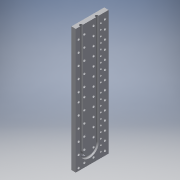
# Autodesk Inventor part: 17-0028-0016
Saved by Autodesk Inventor 2016 SP2 (Build 200236200, 236)
## iProperties
Category: IOP
Company: Universiteit van Amsterdam
RuleStatus: InUse
BeforeDocSave0: Open Form
Created: 2017-11-01
Part Number: 17-0028-0016
Material: Aluminum-6061
Document SubType Name: Modeling
Designer: Daan Giesen
Density: 2.71 g/cm^3
Appearance: Aluminum - Flat - Version 1.1
Mass: 501.104 g
Surface Area: 619.896 cm^2
Volume: 184.909 cm^3
Project: Digital PID Loop
Cost Center: 17-0028
User Status: CNC
Authority: Reichsöllner, Lukas
Description: Heat sink plate
Author: Daan Giesen
Title: Digital PID Loop
Revision Number: A.1
Autodesk Inventor part; units mm, degrees
ref_plane "YZ Plane" through (0, 0, 0) normal (1, 0, 0) x (0, 1, 0)
ref_plane "XZ Plane" through (0, 0, 0) normal (0, 1, 0) x (-1, 0, 0)
ref_plane "XY Plane" through (0, 0, 0) normal (0, 0, 1) x (1, 0, 0)
sketch "Sketch1" plane through (0, 0, 0) normal (0, 0, 1) x (1, 0, 0)
  line L0 (0, 52.5) -> (0, -52.5) construction
  line L1 (-7, 0) -> (7, 0) construction
  line L2 (-5, -37.5) -> (5, -37.5)
  line L3 (5, -37.5) -> (5, 37.5)
  line L4 (5, 37.5) -> (-5, 37.5)
  line L5 (-5, 37.5) -> (-5, -37.5)
  line L6 (-5, -37.5) -> (5, 37.5) construction
  line L7 (5, -37.5) -> (-5, 37.5) construction
  point P0 (0, 0)
  dimension "d0" = 75
  dimension "d1" = 10
  constraints: 12 end point, 2 midpoint, 2 parallel, 1 horizontal, 1 perpendicular
  measures "d0" distance of L2.end L3.end
  measures "d1" distance of L3.end L4.end
extrude "Extrusion1" add sketch "Sketch1" along normal mid plane 284
sketch "Sketch5" plane through (5, -37.5, 142) normal (1, 0, 0) x (0, 0, -1)
  circle A0 centre (154, 67) radius 1.621 projected
  circle A1 centre (154, 41) radius 1.621 projected
  circle A2 centre (174, 67) radius 1.621 projected
  circle A3 centre (174, 41) radius 1.621 projected
  circle A4 centre (194, 67) radius 1.621 projected
  circle A5 centre (194, 41) radius 1.621 projected
  circle A6 centre (214, 67) radius 1.621 projected
  circle A7 centre (214, 41) radius 1.621 projected
  circle A8 centre (234, 67) radius 1.621 projected
  circle A9 centre (234, 41) radius 1.621 projected
  circle A10 centre (254, 67) radius 1.621 projected
  circle A11 centre (254, 41) radius 1.621 projected
  circle A12 centre (274, 67) radius 1.621 projected
  circle A13 centre (274, 41) radius 1.621 projected
  line L0 (299.292, 35) -> (299.292, 75) projected
  line L1 (299.292, 75) -> (0, 75) projected
  line L2 (299.292, 35) -> (0, 35) projected
  circle A14 centre (148, 7) radius 1.621 projected
  circle A15 centre (174, 7) radius 1.621 projected
  circle A16 centre (196.3, 20) radius 1.621 projected
  circle A17 centre (200, 7) radius 1.621 projected
  circle A18 centre (222.3, 20) radius 1.621 projected
  circle A19 centre (226, 7) radius 1.621 projected
  circle A20 centre (248.3, 20) radius 1.621 projected
  circle A21 centre (252, 7) radius 1.621 projected
  circle A22 centre (274.3, 20) radius 1.621 projected
  circle A23 centre (278, 7) radius 1.621 projected
  circle A24 centre (20.3, 13.85) radius 0.7835 projected
  circle A25 centre (33.3, 13.85) radius 0.7835 projected
  circle A26 centre (46.3, 13.85) radius 0.7835 projected
  circle A27 centre (59.3, 13.85) radius 0.7835 projected
  circle A28 centre (72.3, 13.85) radius 0.7835 projected
  circle A29 centre (85.3, 13.85) radius 0.7835 projected
  circle A30 centre (98.3, 13.85) radius 0.7835 projected
  circle A31 centre (111.3, 13.85) radius 0.7835 projected
  circle A32 centre (124.3, 13.85) radius 0.7835 projected
  circle A33 centre (136.7, 25.15) radius 0.7835 projected
  circle A34 centre (157.6, 13.85) radius 0.7835 projected
  circle A35 centre (170.6, 13.85) radius 0.7835 projected
  circle A36 centre (183.6, 13.85) radius 0.7835 projected
  circle A37 centre (196.6, 13.85) radius 0.7835 projected
  circle A38 centre (209, 25.15) radius 0.7835 projected
  circle A39 centre (222.6, 13.85) radius 0.7835 projected
  circle A40 centre (235, 25.15) radius 0.7835 projected
  circle A41 centre (248.6, 13.85) radius 0.7835 projected
  circle A42 centre (261, 25.15) radius 0.7835 projected
  circle A43 centre (274, 25.15) radius 0.7835 projected
  circle A44 centre (261.6, 13.85) radius 0.7835 projected
  circle A45 centre (248, 25.15) radius 0.7835 projected
  circle A46 centre (235.6, 13.85) radius 0.7835 projected
  circle A47 centre (222, 25.15) radius 0.7835 projected
  circle A48 centre (209.6, 13.85) radius 0.7835 projected
  circle A49 centre (196, 25.15) radius 0.7835 projected
  circle A50 centre (170, 25.15) radius 0.7835 projected
  circle A51 centre (144.6, 13.85) radius 0.7835 projected
  circle A52 centre (123.7, 25.15) radius 0.7835 projected
  circle A53 centre (97.7, 25.15) radius 0.7835 projected
  circle A54 centre (71.7, 25.15) radius 0.7835 projected
  circle A55 centre (58.7, 25.15) radius 0.7835 projected
  circle A56 centre (45.7, 25.15) radius 0.7835 projected
  circle A57 centre (32.7, 25.15) radius 0.7835 projected
  circle A58 centre (19.7, 25.15) radius 0.7835 projected
  circle A59 centre (7.3, 13.85) radius 0.7835 projected
  line L3 (289.292, 0) -> (289.292, 30) projected
  line L4 (289.292, 30) -> (0, 30) projected
  line L5 (0, 0) -> (0, 30) projected
  line L6 (289.292, 0) -> (0, 0) projected
  circle A60 centre (84.7, 25.15) radius 0.7835 projected
  circle A61 centre (84.7, 25.15) radius 0.7835 projected
  circle A62 centre (20.3, 20) radius 1.621 projected
  circle A63 centre (24, 7) radius 1.621 projected
  circle A64 centre (46.3, 20) radius 1.621 projected
  circle A65 centre (50, 7) radius 1.621 projected
  circle A66 centre (72.3, 20) radius 1.621 projected
  circle A67 centre (76, 7) radius 1.621 projected
  circle A68 centre (98.3, 20) radius 1.621 projected
  circle A69 centre (102, 7) radius 1.621 projected
  circle A70 centre (124.3, 20) radius 1.621 projected
  circle A71 centre (128, 7) radius 1.621 projected
  circle A72 centre (110.7, 25.15) radius 0.7835 projected
  circle A73 centre (110.7, 25.15) radius 0.7835 projected
  circle A74 centre (144, 20) radius 1.621 projected
  circle A75 centre (144.3, 20) radius 1.621 projected
  circle A76 centre (157, 25.15) radius 0.7835 projected
  circle A77 centre (157, 25.15) radius 0.7835 projected
  circle A78 centre (170, 20) radius 1.621 projected
  circle A79 centre (170.3, 20) radius 1.621 projected
  circle A80 centre (183, 25.15) radius 0.7835 projected
  circle A81 centre (183, 25.15) radius 0.7835 projected
  circle A82 centre (258.35, 57.639) radius 1.6 projected
  circle A83 centre (232.35, 57.639) radius 1.6 projected
  circle A84 centre (206.35, 57.639) radius 1.6 projected
  circle A85 centre (180.35, 57.639) radius 1.6 projected
  circle A86 centre (154.35, 57.639) radius 1.6 projected
  circle A87 centre (167.35, 57.639) radius 1.6 projected
  circle A88 centre (193.35, 57.639) radius 1.6 projected
  circle A89 centre (219.35, 57.639) radius 1.6 projected
  circle A90 centre (245.35, 57.639) radius 1.6 projected
  circle A91 centre (271.35, 57.639) radius 1.6 projected
  circle A92 centre (14, 67) radius 1.621 projected
  circle A93 centre (14, 41) radius 1.621 projected
  circle A94 centre (34, 67) radius 1.621 projected
  circle A95 centre (34, 41) radius 1.621 projected
  circle A96 centre (54, 67) radius 1.621 projected
  circle A97 centre (54, 41) radius 1.621 projected
  circle A98 centre (74, 67) radius 1.621 projected
  circle A99 centre (74, 41) radius 1.621 projected
  circle A100 centre (94, 67) radius 1.621 projected
  circle A101 centre (94, 41) radius 1.621 projected
  circle A102 centre (114, 67) radius 1.621 projected
  circle A103 centre (114, 41) radius 1.621 projected
  circle A104 centre (134, 67) radius 1.621 projected
  circle A105 centre (134, 41) radius 1.621 projected
  circle A106 centre (121.05, 57.639) radius 1.6 projected
  circle A107 centre (95.05, 57.639) radius 1.6 projected
  circle A108 centre (69.05, 57.639) radius 1.6 projected
  circle A109 centre (43.05, 57.639) radius 1.6 projected
  circle A110 centre (17.05, 57.639) radius 1.6 projected
  circle A111 centre (30.05, 57.639) radius 1.6 projected
  circle A112 centre (56.05, 57.639) radius 1.6 projected
  circle A113 centre (82.05, 57.639) radius 1.6 projected
  circle A114 centre (108.05, 57.639) radius 1.6 projected
  circle A115 centre (134.05, 57.639) radius 1.6 projected
  line L7 (0, 35) -> (0, 75) projected
  point P0 (142, 37.5)
  point P1 (274, 67)
  point P2 (254, 67)
  point P3 (274, 41)
  point P4 (194, 67)
  point P5 (174, 67)
  point P6 (174, 41)
  point P7 (154, 41)
  point P8 (134, 67)
  point P9 (134, 41)
  point P10 (114, 41)
  point P11 (94, 41)
  point P12 (94, 67)
  point P13 (54, 67)
  point P14 (34, 41)
  point P15 (34, 67)
  point P16 (14, 67)
  point P17 (274.3, 20)
  point P18 (252, 7)
  point P19 (222.3, 20)
  point P20 (226, 7)
  point P21 (196.3, 20)
  point P22 (200, 7)
  point P23 (144.3, 20)
  point P24 (148, 7)
  point P25 (124.3, 20)
  point P26 (128, 7)
  point P27 (72.3, 20)
  point P28 (76, 7)
  point P29 (24, 7)
  point P30 (20.3, 20)
  constraints: 36 coincident
hole "Hole1" at (5, -17.5, -132.3) at (5, -30.5, -136) at (5, -17.5, -106.3) at (5, -30.5, -110) at (5, -17.5, -80.3) at (5, -30.5, -84) at (5, -17.5, -54.3) at (5, -30.5, -58) at (5, -17.5, -28.3) at (5, -30.5, -32) at (5, -17.5, -2.3) at (5, -30.5, -6) at (5, -17.5, 17.7) at (5, -30.5, 14) at (5, -17.5, 43.7) at (5, -30.5, 40) at (5, -17.5, 69.7) at (5, -30.5, 66) at (5, -17.5, 95.7) at (5, -30.5, 92) at (5, -30.5, 118) at (5, -17.5, 121.7) at (5, 29.5, 128) at (5, 3.5, 128) at (5, 29.5, 108) at (5, 3.5, 108) at (5, 29.5, 88) at (5, 3.5, 88) at (5, 29.5, 68) at (5, 29.5, 48) at (5, 29.5, 28) at (5, 3.5, 68) at (5, 3.5, 48) at (5, 3.5, 28) at (5, 3.5, 8) at (5, 3.5, -12) at (5, 3.5, -32) at (5, 3.5, -52) at (5, 3.5, -72) at (5, 3.5, -92) at (5, 3.5, -112) at (5, 3.5, -132) at (5, 29.5, -132) at (5, 29.5, -112) at (5, 29.5, -92) at (5, 29.5, -72) at (5, 29.5, -52) at (5, 29.5, -32) at (5, 29.5, -12) at (5, 29.5, 8) direction (-1, 0, 0) diameter 5.3 end through all
sketch "Sketch2" plane through (0, 0, 142) normal (0, 0, 1) x (1, 0, 0)
  line L0 (-5, -37.5) -> (5, -37.5) projected
  line L1 (5, -37.5) -> (5, 37.5) projected
  line L2 (5, 37.5) -> (-5, 37.5) projected
  line L3 (-5, 37.5) -> (-5, -37.5) projected
  arc A0 (3, 15) -> (3, 9) centre (3, 12) ccw
  line L4 (5, 15) -> (3, 15)
  line L5 (5, 9) -> (3, 9)
  point P0 (0, 0)
  dimension "d4" = 6
  dimension "d5" = 2
  dimension "d6" = 12
  constraints: 4 end point, 2 horizontal, 2 point on circle, 2 point on line, 2 tangent, 1 centre point
  measures "d4" diameter of A0
  measures "d5" distance from line of L1 A0.centre
  measures "d6" vertical distance of point (0, 0) A0.centre
sketch "Sketch3" plane through (5, -37.5, 142) normal (1, 0, 0) x (0, 0, -1)
  line L0 (0, 49.5) -> (250, 49.5)
  arc A0 (250, 13.5) -> (250, 49.5) centre (250, 31.5) ccw
  line L1 (250, 13.5) -> (0, 13.5)
  line L2 (284, 75) -> (284, 0) projected
  point P0 (142, 37.5)
  dimension "d11" = 36
  dimension "d12" = 34
  constraints: 4 end point, 2 horizontal, 2 point on circle, 2 tangent, 1 centre point
  measures "d11" distance between parallel lines of L0 L1
  measures "d12" distance from line of A0.centre L2
sweep "Sweep1" cut profiles "Sketch2" path "Sketch3" path curves L0 A0 L1 contours L5 A0 L4 L1
sketch "Sketch6" plane through (5, -37.5, -142) normal (1, 0, 0) x (0, 0, -1)
  circle A0 centre (-130, 67) radius 1.621 projected
  circle A1 centre (-130, 41) radius 1.621 projected
  circle A2 centre (-110, 67) radius 1.621 projected
  circle A3 centre (-110, 41) radius 1.621 projected
  circle A4 centre (-90, 67) radius 1.621 projected
  circle A5 centre (-90, 41) radius 1.621 projected
  circle A6 centre (-70, 67) radius 1.621 projected
  circle A7 centre (-70, 41) radius 1.621 projected
  circle A8 centre (-50, 67) radius 1.621 projected
  circle A9 centre (-50, 41) radius 1.621 projected
  circle A10 centre (-30, 67) radius 1.621 projected
  circle A11 centre (-30, 41) radius 1.621 projected
  circle A12 centre (-10, 67) radius 1.621 projected
  circle A13 centre (-10, 41) radius 1.621 projected
  circle A14 centre (-25.65, 57.639) radius 1.6 projected
  circle A15 centre (-51.65, 57.639) radius 1.6 projected
  circle A16 centre (-77.65, 57.639) radius 1.6 projected
  circle A17 centre (-103.65, 57.639) radius 1.6 projected
  circle A18 centre (-129.65, 57.639) radius 1.6 projected
  circle A19 centre (-116.65, 57.639) radius 1.6 projected
  circle A20 centre (-90.65, 57.639) radius 1.6 projected
  circle A21 centre (-64.65, 57.639) radius 1.6 projected
  circle A22 centre (-38.65, 57.639) radius 1.6 projected
  circle A23 centre (-12.65, 57.639) radius 1.6 projected
  line L0 (15.292, 35) -> (15.292, 75) projected
  line L1 (15.292, 75) -> (-284, 75) projected
  line L2 (15.292, 35) -> (-284, 35) projected
  circle A24 centre (-270, 67) radius 1.621 projected
  circle A25 centre (-270, 41) radius 1.621 projected
  circle A26 centre (-250, 67) radius 1.621 projected
  circle A27 centre (-250, 41) radius 1.621 projected
  circle A28 centre (-230, 67) radius 1.621 projected
  circle A29 centre (-230, 41) radius 1.621 projected
  circle A30 centre (-210, 67) radius 1.621 projected
  circle A31 centre (-210, 41) radius 1.621 projected
  circle A32 centre (-190, 67) radius 1.621 projected
  circle A33 centre (-190, 41) radius 1.621 projected
  circle A34 centre (-170, 67) radius 1.621 projected
  circle A35 centre (-170, 41) radius 1.621 projected
  circle A36 centre (-150, 67) radius 1.621 projected
  circle A37 centre (-150, 41) radius 1.621 projected
  circle A38 centre (-162.95, 57.639) radius 1.6 projected
  circle A39 centre (-188.95, 57.639) radius 1.6 projected
  circle A40 centre (-214.95, 57.639) radius 1.6 projected
  circle A41 centre (-240.95, 57.639) radius 1.6 projected
  circle A42 centre (-266.95, 57.639) radius 1.6 projected
  circle A43 centre (-253.95, 57.639) radius 1.6 projected
  circle A44 centre (-227.95, 57.639) radius 1.6 projected
  circle A45 centre (-201.95, 57.639) radius 1.6 projected
  circle A46 centre (-175.95, 57.639) radius 1.6 projected
  circle A47 centre (-149.95, 57.639) radius 1.6 projected
  line L3 (-284, 35) -> (-284, 75) projected
  point P0 (-142, 37.5)
  point P1 (-12.65, 57.639)
  point P2 (-25.65, 57.639)
  point P3 (-38.65, 57.639)
  point P4 (-51.65, 57.639)
  point P5 (-64.65, 57.639)
  point P6 (-77.65, 57.639)
  point P7 (-90.65, 57.639)
  point P8 (-103.65, 57.639)
  point P9 (-116.65, 57.639)
  point P10 (-129.65, 57.639)
  point P11 (-149.95, 57.639)
  point P12 (-162.95, 57.639)
  point P13 (-175.95, 57.639)
  point P14 (-188.95, 57.639)
  point P15 (-201.95, 57.639)
  point P16 (-214.95, 57.639)
  point P17 (-227.95, 57.639)
  point P18 (-240.95, 57.639)
  point P19 (-253.95, 57.639)
  constraints: 10 coincident
hole "Hole2" at (5, 20.139, -129.35) at (5, 20.139, -116.35) at (5, 20.139, -103.35) at (5, 20.139, -90.35) at (5, 20.139, -77.35) at (5, 20.139, -64.35) at (5, 20.139, -51.35) at (5, 20.139, -38.35) at (5, 20.139, -25.35) at (5, 20.139, -12.35) at (5, 20.139, 7.95) at (5, 20.139, 20.95) at (5, 20.139, 33.95) at (5, 20.139, 46.95) at (5, 20.139, 59.95) at (5, 20.139, 72.95) at (5, 20.139, 85.95) at (5, 20.139, 98.95) at (5, 20.139, 111.95) at (5, 20.139, 124.95) direction (-1, 0, 0) diameter 4 end through all
equation "\"d4\" = d4_1"
equation "\"d4_1\" = 6"
body "Solid1"
